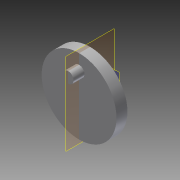
# Autodesk Inventor part: Eccentric
Saved by Autodesk Inventor 2015 (Build 190141000, 141)
## iProperties
Created: 2008-06-07
Part Number: Eccentric
Document SubType Name: Modeling
Designer: tangg
Density: 7.85 g/cm^3
Mass: 10.8718 g
Surface Area: 44.2672 cm^2
Volume: 10.8718 cm^3
Stock Number: Eccentric
Material: Steel
Appearance: Steel
Author: tangg
Autodesk Inventor part; units mm, degrees
ref_plane "XZ Plane" through (0, 0, 0) normal (0, 1, 0) x (-1, 0, 0)
ref_plane "XY Plane" through (0, 0, 0) normal (0, 0, 1) x (1, 0, 0)
sketch "Sketch1" plane through (0, 0, 0) normal (0, 0, 1) x (1, 0, 0)
  circle A0 centre (0, 0) radius 21.7258
  constraints: 1 centre point, 1 coincident
extrude "Extrusion1" add sketch "Sketch1" along normal blind 6.35
sketch "Sketch2" plane through (0, 0, 6.35) normal (0, 0, 1) x (1, 0, 0)
  circle A0 centre (0, 12.7) radius 3.175
  point P0 (0, 0)
  dimension "d4" = 6.35
  constraints: 1 centre point
  measures "d4" diameter of A0
extrude "Extrusion2" add sketch "Sketch2" along normal blind 6.35
sketch "Sketch5" plane through (0, 0, 0) normal (0, 0, -1) x (-1, 0, 0)
  circle A0 centre (0, 0) radius 3.175
  circle A1 centre (0, 0) radius 8.542
  point P0 (0, 0)
  constraints: 2 centre point, 1 coincident
ref_plane "Work Plane3" through (0, 0, -6.35) normal (0, 0, -1) x (-1, 0, 0)
extrude "Extrusion5" add sketch "Sketch5" along normal blind 6.35
sketch "Sketch6" plane through (0, 0, -6.35) normal (0, 0, -1) x (-1, 0, 0)
  circle A0 centre (0, 0) radius 3.175
  spline S0 degree 4 poles (-15.875, 0) (-15.875, 5.123) (-15.6795, 13.2839) (0.7771, 27.615) (13.6923, 12.2077) (15.875, 5.0189) (15.875, 0) knots -1 -1 -1 -1 -1 -0.623021 -0.373021 0 0 0 0 0
  spline S1 degree 4 poles (15.875, 0) (15.875, -4.6644) (10.9112, -18.4609) (-6.6696, -14.611) (-16.1915, -10.8158) (-15.875, 0) knots -1 -1 -1 -1 -1 -0.624992 0 0 0 0 0
  point P0 (0, 0)
  constraints: 2 horizontal alignment, 1 centre point, 4 other
extrude "Extrusion4" [suppressed]
sketch "Sketch7" plane through (0, 0, -12.7) normal (0, 0, -1) x (-1, 0, 0)
  circle A0 centre (0, 0) radius 3.175 projected
  point P0 (0, 0)
  point P1 (15.875, 0)
  point P2 (-15.875, 0)
  constraints: 2 horizontal alignment
body "Solid1"
